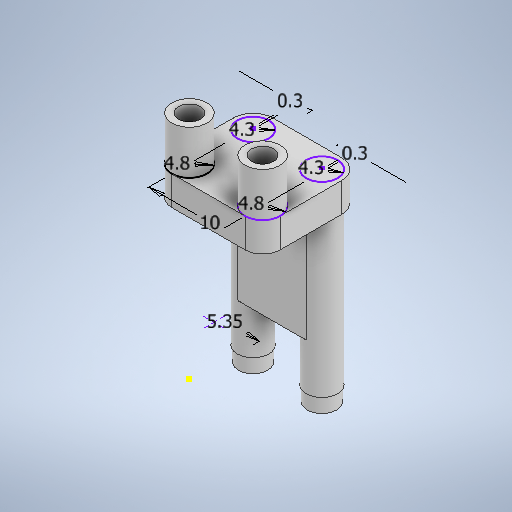
# Autodesk Inventor part: gripper3leftsideservobracket
Saved by Autodesk Inventor 2025.2 (Build 292293000, 293)
## iProperties
Created: 2025-03-30
Part Number: gripper3leftsideservobracket
Material: Generic
Document SubType Name: Modeling
Designer: m_kni
Density: 1 g/cm^3
Appearance: Default
Author: m_kni
## iProperties of the stored document gripper3leftsideservobracket_3DPrint.ipt
Created: 2025-04-02
Part Number: gripper3leftsideservobracket_3DPrint
Material: Generic
Document SubType Name: Modeling
Designer: m_kni
Density: 1 g/cm^3
Appearance: Default
Author: m_kni
Autodesk Inventor part; units mm, degrees
ref_plane "YZ Plane" through (0, 0, 0) normal (1, 0, 0) x (0, 1, 0)
ref_plane "XZ Plane" through (0, 0, 0) normal (0, 1, 0) x (-1, 0, 0)
ref_plane "XY Plane" through (0, 0, 0) normal (0, 0, 1) x (1, 0, 0)
sketch "Sketch1" plane through (0, 0, 0) normal (0, 1, 0) x (-1, 0, 0)
  circle A0 centre (0, 0) radius 2.4
  circle A1 centre (-0.3, -8.4) radius 2.15
  circle A2 centre (-10, 0) radius 2.4
  circle A3 centre (-9.7, -8.4) radius 2.15
  dimension "d0" = 4.8
  dimension "d1" = 4.3
  dimension "d3" = 4.8
  dimension "d4" = 10
  dimension "d5" = 4.3
  dimension "d33" = 0.3
  dimension "d34" = 0.3
  constraints: 4 centre point, 1 coincident
  measures "d0" diameter of A0
  measures "d1" diameter of A1
  measures "d3" diameter of A2
  measures "d4" distance of A2.centre point (0, 0)
  measures "d5" diameter of A3
  measures "d33" horizontal distance of A1.centre point (0, 0)
  measures "d34" horizontal distance of A3.centre A2.centre
extrude "Extrusion1" add sketch "Sketch1" along normal blind 6 contours A0 | A2
sketch "Sketch2" plane through (0, 6, 0) normal (0, 1, 0) x (1, 0, 0)
  circle A0 centre (0, 0) radius 2.4 projected
  circle A1 centre (0, 0) radius 1.5
  circle A2 centre (10, 0) radius 2.4 projected
  circle A3 centre (10, 0) radius 1.5
  dimension "d8" = 3
  dimension "d9" = 3
  constraints: 2 centre point, 2 coincident
  measures "d8" diameter of A1
  measures "d9" diameter of A3
extrude "Extrusion2" cut sketch "Sketch2" against normal blind 4 contours A1 | A3
sketch "Sketch3" plane through (0, 0, 0) normal (0, -1, 0) x (1, 0, 0)
  circle A0 centre (10, 0) radius 2.4 projected
  line L0 (10, 2.4) -> (0, 2.4)
  line L1 (12.4, 0) -> (12.4, -8.4)
  circle A1 centre (0, 0) radius 2.4 projected
  line L2 (-2.4, 0) -> (-2.4, -8.4)
  circle A2 centre (9.7, -8.4) radius 2.15 projected
  circle A3 centre (0.3, -8.4) radius 2.15 projected
  circle A4 centre (0.3, -8.4) radius 2.7
  circle A5 centre (9.7, -8.4) radius 2.7
  line L3 (9.7, -11.1) -> (0.3, -11.1)
  dimension "d12" = 8.4
  dimension "d13" = 8.4
  constraints: 8 end point, 7 point on circle, 2 centre point, 2 coincident, 2 horizontal, 2 tangent, 2 vertical
  measures "d12" distance of L1.start L1.end
  measures "d13" distance of L2.start L2.end
extrude "Extrusion3" add sketch "Sketch3" along normal blind 4 contours A0 | L1 A5 L3 A4 L2 A1 L0 A0 | A5 | A1 | A4 | A2 | A3
extrude "Extrusion4" add sketch "Sketch1" against normal blind 25.5 contours A1 | A3
sketch "Sketch4" plane through (0, -4, 0) normal (0, -1, 0) x (1, 0, 0)
  circle A0 centre (9.7, -8.4) radius 2.15 projected
  line L0 (9.7, -6.25) -> (-0.3, -6.25)
  line L1 (9.7, -10.55) -> (0.3, -10.55)
  circle A1 centre (0.3, -8.4) radius 2.15 projected
  point P0 (0, 0)
  point P1 (0.3, -6.25)
  constraints: 4 end point, 2 horizontal, 2 point on circle, 1 tangent, 2 other
extrude "Extrusion5" add sketch "Sketch4" along normal blind 15.15 contours A0 L1 A1 L0
sketch "Sketch6" plane through (0.3, -25.5, -8.4) normal (0, -1, 0) x (1, 0, 0)
  circle A0 centre (0, 0) radius 1.5 projected
  point P0 (-0.3, 8.4)
  point P1 (-5.35, -0.0027)
  dimension "d24" = 5.35
  measures "d24" distance of point (-5.35, -0.003) A0.centre
sketch "Sketch7" plane through (9.7, -25.5, -8.4) normal (0, -1, 0) x (1, 0, 0)
  circle A0 centre (0, 0) radius 2.15 projected
  circle A1 centre (0, 0) radius 2
  arc A2 (-9.4, 2.15) -> (-9.4, -2.15) centre (-9.4, 0) ccw projected
  circle A3 centre (-9.4, 0) radius 2
  point P0 (-9.7, 8.4)
  dimension "d25" = 4
  dimension "d26" = 4
  constraints: 2 centre point, 2 coincident
  measures "d25" diameter of A1
  measures "d26" diameter of A3
extrude "Extrusion7" add sketch "Sketch7" along normal blind 2 contours A1 | A3
sketch "Sketch8" plane through (0.3, -27.5, -8.4) normal (0, -1, 0) x (1, 0, 0)
  circle A0 centre (0, 0) radius 1.5
  circle A1 centre (9.4, 0) radius 2 projected
  circle A2 centre (9.4, 0) radius 1.5
  point P0 (-0.3, 8.4)
  dimension "d29" = 3
  dimension "d30" = 3
  constraints: 2 centre point, 1 coincident
  measures "d29" diameter of A0
  measures "d30" diameter of A2
extrude "Extrusion8" cut sketch "Sketch8" against normal blind 6 contours A0 | A2
body "Solid1"
